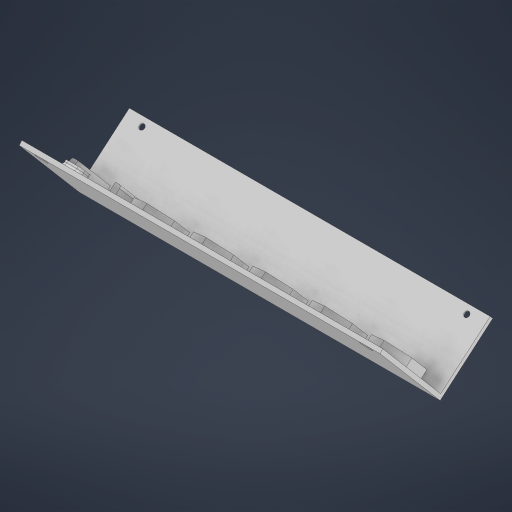
# Autodesk Inventor part: FrontPanel
Saved by Autodesk Inventor 2024 (Build 280153000, 153)
## iProperties
Created: 2023-12-12
Part Number: FrontPanel
Material: Generic
Document SubType Name: Modeling
Designer: Kacper
Density: 1 g/cm^3
Appearance: Default
Author: Kacper
## iProperties of the stored document FrontPanel_3DPrint.ipt
Created: 2023-12-12
Part Number: FrontPanel_3DPrint
Material: Generic
Document SubType Name: Modeling
Designer: Kacper
Density: 1 g/cm^3
Appearance: Default
Author: Kacper
Autodesk Inventor part; units mm, degrees
ref_plane "YZ Plane" through (0, 0, 0) normal (1, 0, 0) x (0, 1, 0)
ref_plane "XZ Plane" through (0, 0, 0) normal (0, 1, 0) x (-1, 0, 0)
ref_plane "XY Plane" through (0, 0, 0) normal (0, 0, 1) x (1, 0, 0)
sketch "Block1" plane through (0, 0, 0) normal (0, 0, 1) x (1, 0, 0)
  arc A0 (12.5237, -32.6294) -> (13.5237, -33.6294) centre (13.5237, -32.6294) ccw
  line L0 (12.5237, -32.6294) -> (12.5237, -30.8294)
  arc A1 (13.5237, -29.8294) -> (12.5237, -30.8294) centre (13.5237, -30.8294) ccw
  line L1 (13.5237, -29.8294) -> (20.6237, -29.8294)
  arc A2 (21.6237, -30.8294) -> (20.6237, -29.8294) centre (20.6237, -30.8294) ccw
  line L2 (21.6237, -30.8294) -> (21.6237, -32.6294)
  arc A3 (20.6237, -33.6294) -> (21.6237, -32.6294) centre (20.6237, -32.6294) ccw
  line L3 (20.6237, -33.6294) -> (13.5237, -33.6294)
  point P0 (17.0737, -31.7294)
sketch "Sketch1" plane through (0, 0, 0) normal (0, 1, 0) x (-1, 0, 0)
  line L0 (90, -17.5) -> (-90, -17.5)
  line L1 (-90, -17.5) -> (-90, 17.5)
  line L2 (-90, 17.5) -> (90, 17.5)
  line L3 (90, 17.5) -> (90, -17.5)
  line L4 (-90, -17.5) -> (90, 17.5) construction
  circle A0 centre (27.74, 0) radius 3.68
  line L5 (80.97, -8.47) -> (55.77, -8.47)
  line L6 (55.77, -8.47) -> (55.77, 8.47)
  line L7 (55.77, 8.47) -> (80.97, 8.47)
  line L8 (80.97, 8.47) -> (80.97, -8.47)
  line L9 (46.74, -17.5) -> (46.74, 17.5) construction
  circle A1 centre (-3.4967, 0) radius 3.68
  circle A2 centre (-34.7333, 0) radius 3.68
  circle A3 centre (-65.97, 0) radius 3.68
  line L10 (27.74, 0) -> (46.74, 0) construction
  line L11 (27.74, 0) -> (-3.4967, 0) construction
  line L12 (-3.4967, 0) -> (-34.7333, 0) construction
  line L13 (-34.7333, 0) -> (-65.97, 0) construction
  line L14 (-65.97, 0) -> (-90, 0) construction
  line L15 (68.37, 8.47) -> (68.37, 14.47) construction
  line L16 (68.37, 14.47) -> (61.37, 14.47)
  line L17 (61.37, 14.47) -> (61.37, 8.47)
  line L18 (68.37, 8.47) -> (75.37, 8.47)
  line L19 (75.37, 8.47) -> (75.37, 14.47)
  line L20 (75.37, 14.47) -> (68.37, 14.47)
  point P0 (0, 0)
  point P1 (0, 0)
  point P2 (55.77, 0)
  dimension "d0" = 180
  dimension "d1" = 35
  dimension "d2" = 7.36
  dimension "d3" = 16.94
  dimension "d4" = 25.2
  dimension "d5" = 9.03
  dimension "d6" = 9.03
  dimension "d7" = 7.36
  dimension "d8" = 7.36
  dimension "d9" = 7.36
  dimension "d10" = 19
  dimension "d11" = 24.03
  dimension "d12" = 6
  dimension "d14" = 7
  dimension "d16" = 7
  dimension "d17" = 6
  constraints: 42 end point, 7 horizontal, 5 midpoint, 5 perpendicular, 4 centre point, 4 parallel, 4 point on line, 2 collinear, 1 coincident, 1 vertical
  measures "d0" distance of L0.start L0.end
  measures "d1" distance of L0.end L1.end
  measures "d2" diameter of A0
  measures "d3" distance of L5.end L6.end
  measures "d4" distance of L5.start L5.end
  measures "d5" distance between parallel lines of L3 L8
  measures "d6" distance between parallel lines of L6 L9
  measures "d7" diameter of A1
  measures "d8" diameter of A2
  measures "d9" diameter of A3
  measures "d10" distance from line of L9 L10.start
  measures "d11" distance of L14.end L13.end
  measures "d12" distance of L15.start L15.end
  measures "d14" distance of L15.end L16.end
  measures "d16" distance of L15.start L18.end
  measures "d17" distance of L18.end L19.end
extrude "Extrusion1" add sketch "Sketch1" against normal blind 2
extrude "Extrusion2" add sketch "Sketch1" against normal blind 0.4 contours L7 L17 L16 L20 L19
sketch "Sketch2" plane through (-90, 0, -17.5) normal (-1, 0, 0) x (0, 0, 1)
  line L0 (35, 0) -> (35, -2) projected
  line L1 (35, 0) -> (42.6604, -6.4279) construction
  line L2 (35, 0) -> (0, 0) projected
  line L3 (0, 0) -> (35, 0) projected
  line L4 (0, 0) -> (-17.5094, -20.8669)
  line L5 (0, 0) -> (0, -2) projected
  line L6 (42.6604, -6.4279) -> (41.5188, -7.7688) construction
  line L7 (10.2473, -44.4987) -> (-17.5094, -20.8669)
  line L8 (35, 0) -> (41.5188, -7.7688)
  line L9 (41.5188, -7.7688) -> (10.2473, -44.4987)
  line L10 (1.5321, -1.2856) -> (-14.7009, -20.6314)
  line L11 (-14.7009, -20.6314) -> (10.021, -41.6794)
  line L12 (10.021, -41.6794) -> (38.9001, -7.7594)
  line L13 (38.9001, -7.7594) -> (33.4679, -1.2856)
  line L14 (35, -2) -> (0, -2) projected
  line L15 (-14.7009, -20.6314) -> (-15.9975, -22.1542)
  line L16 (38.9001, -7.7594) -> (40.2039, -9.3132)
  point P0 (17.5, 0)
  point P1 (34.0674, -2)
  point P2 (0.9326, -2)
  dimension "d22" = 50
  dimension "d23" = 40
  dimension "d24" = 50
  dimension "d25" = 10
  dimension "d27" = 40
  dimension "d28" = 2
  constraints: 24 end point, 4 perpendicular, 2 point on line, 1 collinear, 3 other
  measures "d22" angle of L0 L1
  measures "d23" angle of L4 L5
  measures "d24" distance of L1.end L7.start
  measures "d25" distance of L0.start L1.end
  measures "d27" angle of L0 L8
  measures "d28" distance between parallel lines of L9 L12
extrude "Extrusion3" add sketch "Sketch2" against normal up to surface (180 mm away) contours L8 L9 L16 L13 L14 L0 | L5 L14 L10 L15 L7 L4
extrude "Extrusion4" add sketch "Sketch2" against normal up to surface (180 mm away) separate body contours L9 L7 L15 L11 L12 L16
sketch "Sketch3" plane through (-90, -2, -16.5674) normal (0, -0.6427876, 0.7660444) x (1, 0, 0)
  line L0 (0, -24.3215) -> (180, -24.3215) projected
  line L1 (174, -24.3215) -> (168, -24.3215)
  line L2 (168, -24.3215) -> (168, -20.3215)
  line L3 (168, -20.3215) -> (174, -20.3215)
  line L4 (174, -20.3215) -> (174, -24.3215)
  line L5 (180, -24.3215) -> (180, 0) projected
  line L6 (90, -24.3215) -> (90, -19) construction
  line L7 (12, -24.3215) -> (12, -20.3215)
  line L8 (12, -20.3215) -> (6, -20.3215)
  line L9 (6, -20.3215) -> (6, -24.3215)
  point P0 (90, 12.1814)
  point P1 (12, -24.3215)
  point P2 (168, -24.3215)
  dimension "d33" = 4
  dimension "d34" = 6
  dimension "d35" = 6
  constraints: 16 end point, 4 symmetric about line, 2 parallel, 1 horizontal, 1 midpoint, 1 perpendicular, 1 point on line, 1 vertical
  measures "d33" distance of L1.end L2.end
  measures "d34" distance of L2.end L3.end
  measures "d35" distance between parallel lines of L5 L4
extrude "Extrusion5" add sketch "Sketch3" along normal blind 7 bodies 1
chamfer "Chamfer1" distance 7 angle 45 2 edges at (81, -17.5672, -29.6298) (-81, -17.5672, -29.6298)
sketch "Sketch4" plane through (-84, -20.6314, -32.2009) normal (0, -0.7660444, -0.6427876) x (1, 0, 0)
  line L0 (0, 0) -> (6, 0) projected
  line L1 (6, 0) -> (6, 7) projected
  line L2 (0, 7) -> (6, 7) projected
  line L3 (0, 0) -> (0, 7) projected
  line L4 (162, 0) -> (168, 0) projected
  line L5 (168, 0) -> (168, 7) projected
  line L6 (162, 7) -> (168, 7) projected
  line L7 (162, 0) -> (162, 7) projected
  line L8 (6, 7) -> (0, 0) construction
  circle A0 centre (3, 3.5) radius 1.3
  line L9 (168, 7) -> (162, 0) construction
  circle A1 centre (165, 3.5) radius 1.3
  point P0 (84, 11.4058)
  dimension "d41" = 2.6
  dimension "d42" = 2.6
  constraints: 4 end point, 2 centre point, 2 midpoint
  measures "d41" diameter of A0
  measures "d42" diameter of A1
extrude "Extrusion6" cut sketch "Sketch4" against normal blind 9.25 contours A0 | A1 bodies 1
sketch "Sketch5" plane through (90, 0, -17.5) normal (0, 0.6427876, -0.7660444) x (-1, 0, 0)
  circle A0 centre (51, -13.0934) radius 8.3
  line L0 (0, -25.2541) -> (0, -0.9326) projected
  line L1 (0, -13.0934) -> (180, -13.0934) construction
  line L2 (180, -25.2541) -> (180, -0.9326) projected
  circle A1 centre (24, -13.0934) radius 8.3
  point P0 (90, 11.2488)
  dimension "d45" = 16.6
  dimension "d46" = 16.6
  dimension "d47" = 27
  dimension "d48" = 24
  constraints: 2 centre point, 2 end point, 2 midpoint, 2 point on line
  measures "d45" diameter of A0
  measures "d46" diameter of A1
  measures "d47" distance of A1.centre A0.centre
  measures "d48" distance from line of L0 A1.centre
extrude "Extrusion7" cut sketch "Sketch5" against normal blind 9.25 bodies 1
ref_plane "Work Plane1" through (-84, -20.6314, -32.2009) normal (-1, 0, 0) x (0, -0.6427876, 0.7660444)
sketch "Sketch9" plane through (-84, -20.6314, -32.2009) normal (-1, 0, 0) x (0, -0.6427876, 0.7660444)
  line L0 (25.3827, 45.6201) -> (34.7844, 43.9623) projected
  line L1 (32.7869, 44.3146) -> (32.7367, 37.3147)
  line L2 (34.7844, 43.9623) -> (34.7989, 45.9906) projected
  line L3 (32.7367, 37.3147) -> (28.7367, 37.3147)
  line L4 (28.7367, 37.3147) -> (28.7367, 45.0287)
  point P0 (11.4058, 36.5029)
  dimension "d62" = 7
  dimension "d63" = 4
  constraints: 6 end point, 1 horizontal, 1 parallel, 1 perpendicular, 1 point on line
  measures "d62" distance of L1.start L1.end
  measures "d63" distance of L1.end L3.end
extrude "Extrusion11" add sketch "Sketch9" against normal up to surface (6 mm away) bodies 1
ref_plane "Work Plane2" through (78, -20.6314, -32.2009) normal (-1, 0, 0) x (0, -0.6427876, 0.7660444)
sketch "Sketch10" plane through (78, -20.6314, -32.2009) normal (-1, 0, 0) x (0, -0.6427876, 0.7660444)
  line L0 (32.7367, 37.3147) -> (32.7869, 44.3146) projected
  line L1 (28.7367, 45.0287) -> (32.7869, 44.3146) projected
  line L2 (28.7367, 45.0287) -> (28.7367, 37.3147) projected
  line L3 (28.7367, 37.3147) -> (32.7367, 37.3147) projected
  point P0 (11.4058, 36.5029)
extrude "Extrusion12" add sketch "Sketch10" against normal up to surface (6 mm away) bodies 1
chamfer "Chamfer3" distance 3.25 distance2 7.5 2 edges at (81, -4.6089, 18.7565) (-81, -4.6089, 18.7565) measured on face at (81, -4.2259, 18.4351) measured on face at (-81, -4.2259, 18.4351)
sketch "Sketch11" plane through (-84, -7.7594, 21.4001) normal (0, -0.6482624, 0.761417) x (1, 0, 0)
  line L0 (6, -7) -> (6, 0) projected
  line L1 (0, 0) -> (6, 0) projected
  line L2 (0, -7) -> (0, 0) projected
  line L3 (0, -7) -> (6, -7) projected
  line L4 (168, 0) -> (168, -7) projected
  line L5 (162, 0) -> (168, 0) projected
  line L6 (162, -7) -> (162, 0) projected
  line L7 (162, -7) -> (168, -7) projected
  circle A0 centre (165, -3.5) radius 1.3
  line L8 (0, -7) -> (6, 0) construction
  circle A1 centre (3, -3.5) radius 1.3
  point P0 (84, -7.9647)
  dimension "d72" = 2.6
  dimension "d73" = 2.6
  constraints: 2 centre point, 2 end point, 1 midpoint
  measures "d72" diameter of A0
  measures "d73" diameter of A1
extrude "Extrusion13" cut sketch "Sketch11" against normal blind 10 contours A0 | A1 bodies 1
sketch "Sketch6" plane through (90, 0, 17.5) normal (1, 0, 0) x (0, 0, -1)
  line L0 (0, 0) -> (35, 0) projected
  line L1 (-6.5188, -7.7688) -> (0, 0) projected
  line L2 (-5.2039, -9.3132) -> (-6.5188, -7.7688) projected
  line L3 (0.9326, -2) -> (-5.2039, -9.3132) projected
  line L4 (34.0674, -2) -> (0.9326, -2) projected
  line L5 (49.7009, -20.6314) -> (34.0674, -2) projected
  line L6 (50.9975, -22.1542) -> (49.7009, -20.6314) projected
  line L7 (52.5094, -20.8669) -> (50.9975, -22.1542) projected
  line L8 (35, 0) -> (52.5094, -20.8669) projected
  line L9 (49.7009, -20.6314) -> (50.9975, -22.1542) projected
  line L10 (24.979, -41.6794) -> (49.7009, -20.6314) projected
  line L11 (-3.9001, -7.7594) -> (24.979, -41.6794) projected
  line L12 (-5.2039, -9.3132) -> (-3.9001, -7.7594) projected
  line L13 (24.7527, -44.4987) -> (-5.2039, -9.3132) projected
  line L14 (50.9975, -22.1542) -> (24.7527, -44.4987) projected
  point P0 (17.5, 0)
extrude "Extrusion8" add sketch "Sketch6" along normal blind 2 bodies 1
sketch "Sketch7" plane through (-90, 0, -17.5) normal (-1, 0, 0) x (0, 0, 1)
  line L0 (10.021, -41.6794) -> (-14.7009, -20.6314) projected
  line L1 (-14.7009, -20.6314) -> (-15.9975, -22.1542) projected
  line L2 (-15.9975, -22.1542) -> (10.2473, -44.4987) projected
  line L3 (10.2473, -44.4987) -> (40.2039, -9.3132) projected
  line L4 (40.2039, -9.3132) -> (38.9001, -7.7594) projected
  line L5 (38.9001, -7.7594) -> (10.021, -41.6794) projected
  line L6 (0, 0) -> (35, 0) projected
  line L7 (0, 0) -> (-17.5094, -20.8669) projected
  line L8 (-17.5094, -20.8669) -> (-15.9975, -22.1542) projected
  line L9 (-15.9975, -22.1542) -> (-14.7009, -20.6314) projected
  line L10 (-14.7009, -20.6314) -> (0.9326, -2) projected
  line L11 (34.0674, -2) -> (0.9326, -2) projected
  line L12 (34.0674, -2) -> (40.2039, -9.3132) projected
  line L13 (40.2039, -9.3132) -> (41.5188, -7.7688) projected
  line L14 (41.5188, -7.7688) -> (35, 0) projected
  point P0 (17.5, 0)
extrude "Extrusion9" add sketch "Sketch7" along normal blind 2 bodies 1
sketch "Sketch8" plane through (-90, -44.4987, -7.2527) normal (0, -0.761417, -0.6482624) x (1, 0, 0)
  ellipse E0 centre (9, -30.9684) end of major axis (10.3, -30.9684) minor radius 1.3 projected
  ellipse E1 centre (171, -30.9684) end of major axis (172.3, -30.9684) minor radius 1.3 projected
  point P0 (90, -23.3245)
extrude "Extrusion10" cut sketch "Sketch8" against normal blind 2 bodies 2
sketch "Sketch12" plane through (-90, -9.3132, 22.7039) normal (0, -0.6482624, 0.761417) x (1, 0, 0)
  circle A0 centre (9, -3.1621) radius 1.3 projected
  circle A1 centre (171, -3.1621) radius 1.3 projected
  point P0 (90, -7.6268)
extrude "Extrusion14" cut sketch "Sketch12" against normal blind 10 bodies 2
chamfer "Chamfer2" distance 1.5 angle 45 4 edges at (-82.3, -24.423, -30.8326) (79.7, -24.423, -30.8326) (79.7, -11.7209, 20.654) (-82.3, -11.7209, 20.654)
sketch "Sketch13" plane through (90, -41.6794, -7.479) normal (0, 0.6482624, -0.761417) x (-1, 0, 0)
  ellipse E0 centre (24.03, 36.5837) end of major axis (20.35, 36.5837) minor radius 2.3856 projected
  ellipse E1 centre (55.2667, 36.5837) end of major axis (51.5867, 36.5837) minor radius 2.3856 projected
  ellipse E2 centre (86.5033, 36.5837) end of major axis (82.8233, 36.5837) minor radius 2.3856 projected
  ellipse E3 centre (117.74, 36.5837) end of major axis (114.06, 36.5837) minor radius 2.3856 projected
  line L0 (19.65, 13.5833) -> (12, 9.1665)
  line L1 (12, 9.1665) -> (4.35, 13.5833)
  line L2 (4.35, 13.5833) -> (4.35, 22.4167)
  line L3 (4.35, 22.4167) -> (12, 26.8335)
  line L4 (12, 26.8335) -> (19.65, 22.4167)
  line L5 (19.65, 22.4167) -> (19.65, 13.5833)
  line L6 (12, 18) -> (0, 18) construction
  line L7 (49.25, 13.5833) -> (41.6, 9.1665)
  line L8 (41.6, 9.1665) -> (33.95, 13.5833)
  line L9 (33.95, 13.5833) -> (33.95, 22.4167)
  line L10 (33.95, 22.4167) -> (41.6, 26.8335)
  line L11 (41.6, 26.8335) -> (49.25, 22.4167)
  line L12 (49.25, 22.4167) -> (49.25, 13.5833)
  line L13 (41.6, 18) -> (12, 18) construction
  line L14 (78.85, 13.5833) -> (71.2, 9.1665)
  line L15 (71.2, 9.1665) -> (63.55, 13.5833)
  line L16 (63.55, 13.5833) -> (63.55, 22.4167)
  line L17 (63.55, 22.4167) -> (71.2, 26.8335)
  line L18 (71.2, 26.8335) -> (78.85, 22.4167)
  line L19 (78.85, 22.4167) -> (78.85, 13.5833)
  line L20 (71.2, 18) -> (41.6, 18) construction
  line L21 (108.45, 13.5833) -> (100.8, 9.1665)
  line L22 (100.8, 9.1665) -> (93.15, 13.5833)
  line L23 (93.15, 13.5833) -> (93.15, 22.4167)
  line L24 (93.15, 22.4167) -> (100.8, 26.8335)
  line L25 (100.8, 26.8335) -> (108.45, 22.4167)
  line L26 (108.45, 22.4167) -> (108.45, 13.5833)
  line L27 (100.8, 18) -> (71.2, 18) construction
  line L28 (138.05, 13.5833) -> (130.4, 9.1665)
  line L29 (130.4, 9.1665) -> (122.75, 13.5833)
  line L30 (122.75, 13.5833) -> (122.75, 22.4167)
  line L31 (122.75, 22.4167) -> (130.4, 26.8335)
  line L32 (130.4, 26.8335) -> (138.05, 22.4167)
  line L33 (138.05, 22.4167) -> (138.05, 13.5833)
  line L34 (130.4, 18) -> (100.8, 18) construction
  line L35 (167.65, 13.5833) -> (160, 9.1665)
  line L36 (160, 9.1665) -> (152.35, 13.5833)
  line L37 (152.35, 13.5833) -> (152.35, 22.4167)
  line L38 (152.35, 22.4167) -> (160, 26.8335)
  line L39 (160, 26.8335) -> (167.65, 22.4167)
  line L40 (167.65, 22.4167) -> (167.65, 13.5833)
  line L41 (160, 18) -> (130.4, 18) construction
  line L42 (180, 44.5485) -> (180, 0) projected
  line L43 (180, 18) -> (160, 18) construction
  line L44 (0, 44.5485) -> (0, 0) projected
  line L45 (12, 6.3953) -> (22.05, 12.1976)
  line L46 (22.05, 12.1976) -> (22.05, 23.8024)
  line L47 (22.05, 23.8024) -> (12, 29.6047)
  line L48 (12, 29.6047) -> (1.95, 23.8024)
  line L49 (1.95, 23.8024) -> (1.95, 12.1976)
  line L50 (1.95, 12.1976) -> (12, 6.3953)
  line L51 (31.55, 12.1976) -> (41.6, 6.3953)
  line L52 (41.6, 6.3953) -> (51.65, 12.1976)
  line L53 (51.65, 12.1976) -> (51.65, 23.8024)
  line L54 (51.65, 23.8024) -> (41.6, 29.6047)
  line L55 (41.6, 29.6047) -> (31.55, 23.8024)
  line L56 (31.55, 23.8024) -> (31.55, 12.1976)
  line L57 (61.15, 12.1976) -> (71.2, 6.3953)
  line L58 (71.2, 6.3953) -> (81.25, 12.1976)
  line L59 (81.25, 12.1976) -> (81.25, 23.8024)
  line L60 (81.25, 23.8024) -> (71.2, 29.6047)
  line L61 (71.2, 29.6047) -> (61.15, 23.8024)
  line L62 (61.15, 23.8024) -> (61.15, 12.1976)
  line L63 (90.75, 12.1976) -> (100.8, 6.3953)
  line L64 (100.8, 6.3953) -> (110.85, 12.1976)
  line L65 (110.85, 12.1976) -> (110.85, 23.8024)
  line L66 (110.85, 23.8024) -> (100.8, 29.6047)
  line L67 (100.8, 29.6047) -> (90.75, 23.8024)
  line L68 (90.75, 23.8024) -> (90.75, 12.1976)
  line L69 (120.35, 12.1976) -> (130.4, 6.3953)
  line L70 (130.4, 6.3953) -> (140.45, 12.1976)
  line L71 (140.45, 12.1976) -> (140.45, 23.8024)
  line L72 (140.45, 23.8024) -> (130.4, 29.6047)
  line L73 (130.4, 29.6047) -> (120.35, 23.8024)
  line L74 (120.35, 23.8024) -> (120.35, 12.1976)
  line L75 (149.95, 12.1976) -> (160, 6.3953)
  line L76 (160, 6.3953) -> (170.05, 12.1976)
  line L77 (170.05, 12.1976) -> (170.05, 23.8024)
  line L78 (170.05, 23.8024) -> (160, 29.6047)
  line L79 (160, 29.6047) -> (149.95, 23.8024)
  line L80 (149.95, 23.8024) -> (149.95, 12.1976)
  point P0 (90, 36.5837)
  dimension "d79" = 15.3
  dimension "d80" = 15.3
  dimension "d81" = 15.3
  dimension "d82" = 15.3
  dimension "d83" = 15.3
  dimension "d84" = 15.3
  dimension "d85" = 12
  dimension "d86" = 2.4
  dimension "d87" = 2.4
  dimension "d88" = 2.4
  dimension "d89" = 2.4
  dimension "d90" = 2.4
  dimension "d91" = 2.4
  constraints: 158 end point, 6 horizontal, 6 vertical, 5 collinear, 2 point on line, 1 perpendicular, 112 other
  measures "d79" distance between parallel lines of L2 L5
  measures "d80" distance between parallel lines of L9 L12
  measures "d81" distance between parallel lines of L16 L19
  measures "d82" distance between parallel lines of L23 L26
  measures "d83" distance between parallel lines of L30 L33
  measures "d84" distance between parallel lines of L37 L40
  measures "d85" distance of L6.start L6.end
  measures "d86" distance between parallel lines of L0 L45
  measures "d87" distance between parallel lines of L8 L51
  measures "d88" distance between parallel lines of L15 L57
  measures "d89" distance between parallel lines of L22 L63
  measures "d90" distance between parallel lines of L29 L69
  measures "d91" distance between parallel lines of L36 L75
extrude "Extrusion15" add sketch "Sketch13" along normal blind 4 contours L50 L49 L48 L47 L46 L45 | L56 L55 L54 L53 L52 L51 | L62 L61 L60 L59 L58 L57 | L68 L67 L66 L65 L64 L63 | L74 L73 L72 L71 L70 L69 bodies 2
sketch "Sketch14" plane through (90, -41.6794, -7.479) normal (0, 0.6482624, -0.761417) x (-1, 0, 0)
  line L0 (170, 2.3885) -> (148.28, 2.3885)
  line L1 (148.28, 2.3885) -> (148.28, 37.4885)
  line L2 (148.28, 37.4885) -> (170, 37.4885)
  line L3 (170, 37.4885) -> (170, 2.3885)
  line L4 (145.28, 2.3885) -> (167, 2.3885)
  line L5 (167, 2.3885) -> (167, 37.4885)
  line L6 (167, 37.4885) -> (145.28, 37.4885)
  line L7 (145.28, 37.4885) -> (145.28, 2.3885)
  line L8 (180, 0) -> (0, 0) projected
  line L9 (170, 37.4885) -> (145.28, 37.4885)
  line L10 (162.14, 37.4885) -> (153.14, 37.4885)
  line L11 (153.14, 37.4885) -> (153.14, 42)
  line L12 (153.14, 42) -> (162.14, 42)
  line L13 (162.14, 42) -> (162.14, 37.4885)
  line L14 (162.14, 37.4885) -> (162.14, 34.4885)
  line L15 (162.14, 34.4885) -> (153.14, 34.4885)
  line L16 (153.14, 34.4885) -> (153.14, 37.4885)
  line L17 (167, 34.4885) -> (162.14, 34.4885)
  line L18 (153.14, 34.4885) -> (148.28, 34.4885)
  line L19 (151.14, 34.4885) -> (151.14, 2.3885)
  line L20 (164.14, 34.4885) -> (164.14, 2.3885)
  line L21 (148.28, 30) -> (151.14, 30) construction
  line L22 (164.14, 30) -> (167, 30) construction
  line L23 (180, 44.5485) -> (180, 0) projected
  line L24 (170, 27.4885) -> (167, 27.4885)
  line L25 (148.28, 27.4885) -> (145.28, 27.4885)
  point P0 (90, 36.5837)
  point P1 (170, 19.9385)
  point P2 (151.14, 2.3885)
  point P3 (164.14, 2.3885)
  point P4 (153.14, 37.4885)
  point P5 (153.14, 37.4885)
  point P6 (162.14, 37.4885)
  point P7 (167, 2.3885)
  point P8 (146.78, 27.4885)
  dimension "d95" = 3
  dimension "d96" = 3
  dimension "d97" = 18.72
  dimension "d98" = 2.3885
  dimension "d99" = 35.1
  dimension "d100" = 9
  dimension "d101" = 3
  dimension "d104" = 13
  dimension "d117" = 10
  dimension "d120" = 10
  constraints: 48 end point, 21 point on line, 8 perpendicular, 6 horizontal, 6 parallel, 3 collinear, 2 midpoint, 1 vertical
  measures "d95" distance from line of point (170, 19.938) L5
  measures "d96" distance between parallel lines of L7 L1
  measures "d97" distance between parallel lines of L1 L5
  measures "d98" distance between parallel lines of L8 L0
  measures "d99" distance of L6.end L4.start
  measures "d100" distance of L11.end L12.end
  measures "d101" distance of L10.start L14.end
  measures "d104" distance between parallel lines of L19 L20
  measures "d117" distance between parallel lines of L23 L3
  measures "d120" distance from line of L9 point (146.78, 27.488)
extrude "Extrusion16" cut sketch "Sketch14" against normal blind 1 from surface at 0 contours L0 L19 L18 L15 L17 L20 bodies 2
extrude "Extrusion17" add sketch "Sketch14" along normal blind 2.2 contours L15 L16 L2 L14 | L2 L11 L12 L13 bodies 2
sketch "Sketch15" plane through (90, -40.2532, -9.1541) normal (0, 0.6482624, -0.761417) x (-1, 0, 0)
  line L0 (167, 37.4885) -> (145.28, 37.4885) projected
  line L1 (162.14, 34.4885) -> (162.14, 42) projected
  line L2 (162.14, 42) -> (153.14, 42) projected
  line L3 (153.14, 42) -> (153.14, 34.4885) projected
  line L4 (153.14, 34.4885) -> (162.14, 34.4885) projected
  line L5 (151, 35.7885) -> (167, 35.7885)
  point P0 (90, 36.5837)
  point P1 (153.14, 37.4885)
  point P2 (162.14, 37.4885)
  point P3 (153.14, 35.7885)
  point P4 (162.14, 35.7885)
  dimension "d126" = 1.7
  constraints: 2 end point, 1 horizontal
  measures "d126" distance between parallel lines of L0 L5
extrude "Extrusion18" add sketch "Sketch15" along normal blind 1.7 separate body contours L1 L5 L3 L0 | L0 L3 L2 L1
extrude "Extrusion21" add sketch "Sketch14" along normal blind 5.1 contours L0 L5 L24 L3 | L4 L7 L25 L1 bodies 2
sketch "Sketch16" plane through (90, -39.1511, -10.4485) normal (0, 0.6482624, -0.761417) x (-1, 0, 0)
  line L0 (153.14, 42) -> (153.14, 35.7885) projected
  line L1 (162.14, 35.7885) -> (162.14, 42) projected
  line L2 (162.14, 42) -> (153.14, 42) projected
  line L3 (162.14, 34.4885) -> (162.14, 42) projected
  line L4 (153.14, 42) -> (153.14, 34.4885) projected
  line L5 (153.14, 34.4885) -> (162.14, 34.4885) projected
  circle A0 centre (157.64, 39.7442) radius 1.7
  line L6 (162.14, 42) -> (153.14, 42) projected
  line L7 (153.14, 35.7885) -> (162.14, 35.7885) projected
  point P0 (90, 36.5837)
  dimension "d109" = 3.4
  constraints: 1 centre point
  measures "d109" diameter of A0
extrude "Extrusion19" add sketch "Sketch16" along normal blind 1.7 bodies 3
fillet "Fillet1" radius 2 12 edges at (-72.14, -8.9868, 18.9105) (-63.14, -8.9868, 18.9105) (-63.14, -14.7061, 14.0411) (-72.14, -14.7061, 14.0411) (-74.14, -27.64, 4.474) (-61.14, -27.64, 4.474) (-61.14, -28.2895, 5.2369) (-74.14, -28.2895, 5.2369) (-63.14, -7.1716, 16.7785) (-72.14, -7.1716, 16.7785) (-63.14, -12.34, 11.2619) (-72.14, -12.34, 11.2619)
sketch "Sketch17" plane through (-90, -20.6314, -32.2009) normal (0, 0.761417, 0.6482624) x (1, 0, 0)
  line L0 (14.9463, -32.4684) -> (29.7737, -32.4684) projected
  line L1 (22.36, -33.4684) -> (22.36, -31.4684) construction
  arc A0 (17.81, -32.4684) -> (18.81, -33.4684) centre (18.81, -32.4684) ccw
  line L2 (17.81, -32.4684) -> (17.81, -30.6684)
  arc A1 (18.81, -29.6684) -> (17.81, -30.6684) centre (18.81, -30.6684) ccw
  line L3 (18.81, -29.6684) -> (25.91, -29.6684)
  arc A2 (26.91, -30.6684) -> (25.91, -29.6684) centre (25.91, -30.6684) ccw
  line L4 (26.91, -30.6684) -> (26.91, -32.4684)
  arc A3 (25.91, -33.4684) -> (26.91, -32.4684) centre (25.91, -32.4684) ccw
  line L5 (25.91, -33.4684) -> (18.81, -33.4684)
  point P0 (90, -11.1438)
  point P1 (22.36, -32.4684)
  dimension "d114" = 1
  constraints: 2 end point, 2 midpoint, 1 vertical, 1 other
  measures "d114" distance from line of L0 L1.start
extrude "Extrusion20" cut sketch "Sketch17" along normal mid plane 13.95 bodies 2
fillet "Fillet2" radius 1.25 13 edges at (-78.5, -20.7492, 10.3408) (-80, -30.3049, 2.2051) (-80, -26.9988, -1.6781) (-55.28, -26.9988, -1.6781) (-56.78, -20.7492, 10.3408) (-55.28, -30.3049, 2.2051) (-63.7258, -10.1459, 19.3683) (-67.64, -9.6999, 19.748) (-71.5542, -10.1459, 19.3683) (-72.14, -12.5595, 17.3133) (-71.5542, -14.9732, 15.2584) (-63.7258, -14.9732, 15.2584) (-63.14, -12.5595, 17.3133)
extrude "Extrusion22" cut sketch "Sketch16" against normal blind 4.9 contours A0 bodies 2
sketch "Sketch18" plane through (90, -38.0491, -11.7429) normal (0, 0.6482624, -0.761417) x (-1, 0, 0)
  circle A0 centre (157.64, 39.7442) radius 1.7 projected
  point P0 (90, 36.5837)
extrude "Extrusion23" cut sketch "Sketch18" against normal through all bodies 3
equation "\"d6\" = d5"
equation "\"d7\" = d2"
equation "\"d8\" = d2"
equation "\"d9\" = d2"
equation "\"d42\" = d41"
equation "\"d46\" = d45"
equation "\"d79\" = d80"
equation "\"d80\" = d81"
equation "\"d81\" = d82"
equation "\"d82\" = d83"
equation "\"d83\" = d84"
equation "\"d96\" = d95"
body "Solid1"
body "Solid4"
